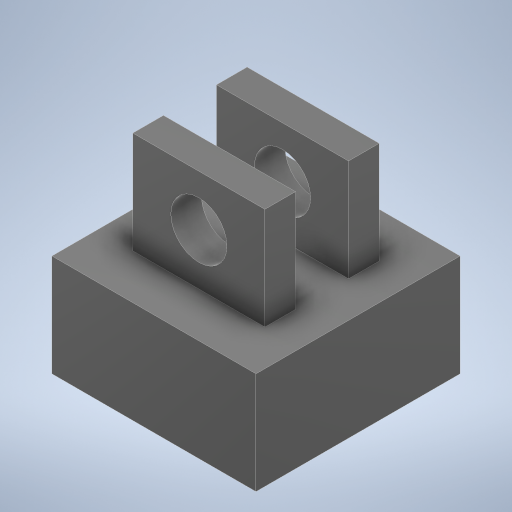
# Autodesk Inventor part: RollZ
Saved by Autodesk Inventor 2023 (Build 270158000, 158)
## iProperties
Created: 2023-10-26
Part Number: RollZ
Material: Thermoplastic Resin
Document SubType Name: Modeling
Designer: Mustapha
Density: 1.28 g/cm^3
Appearance: Smooth - Black
Mass: 5.5597 g
Surface Area: 24.3284 cm^2
Volume: 4.34352 cm^3
Author: Mustapha
Autodesk Inventor part; units mm, degrees
ref_plane "YZ Plane" through (0, 0, 0) normal (1, 0, 0) x (0, 1, 0)
ref_plane "XZ Plane" through (0, 0, 0) normal (0, 1, 0) x (-1, 0, 0)
ref_plane "XY Plane" through (0, 0, 0) normal (0, 0, 1) x (1, 0, 0)
sketch "Sketch1" plane through (0, 0, 0) normal (0, 1, 0) x (-1, 0, 0)
  line L0 (0, 0) -> (20, 0)
  line L1 (20, 0) -> (20, -20)
  line L2 (20, -20) -> (0, -20)
  line L3 (0, -20) -> (0, 0)
  point P0 (0, -10)
  point P1 (20, -10)
  dimension "d0" = 20
  dimension "d1" = 20
  constraints: 8 end point, 2 midpoint, 2 parallel, 1 horizontal, 1 perpendicular
  measures "d0" distance between parallel lines of L2 L0
  measures "d1" distance of point (0, -10) point (20, -10)
extrude "Extrusion1" add sketch "Sketch1" along normal blind 10
sketch "Sketch2" plane through (0, 0, 0) normal (0, -1, 0) x (1, 0, 0)
  circle A0 centre (-10, -10) radius 2.1511
  line L0 (-20, 0) -> (0, 0) projected
  line L1 (-13.8262, -12.1511) -> (-13.776, -7.7619)
  line L2 (-13.776, -7.7619) -> (-9.9498, -5.6108)
  line L3 (-9.9498, -5.6108) -> (-6.1738, -7.8489)
  line L4 (-6.1738, -7.8489) -> (-6.224, -12.2381)
  line L5 (-6.224, -12.2381) -> (-10.0502, -14.3892)
  line L6 (-10.0502, -14.3892) -> (-13.8262, -12.1511)
  dimension "d4" = 10
  constraints: 12 end point, 1 centre point, 1 coincident, 13 other
  measures "d4" distance from line of L0 A0.centre
extrude "Extrusion2" cut sketch "Sketch2" against normal blind 1 contours A0 | L1 L2 L3 L4 L5 L6
sketch "Sketch3" plane through (0, 1, 0) normal (0, -1, 0) x (1, 0, 0)
  circle A0 centre (-9.9498, -10) radius 3
  line L0 (-20, 0) -> (0, 0) projected
  point P0 (-10, 0)
  dimension "d7" = 6
  dimension "d8" = 10
  constraints: 1 centre point, 1 midpoint
  measures "d7" diameter of A0
  measures "d8" vertical distance of point (-10, 0) A0.centre
extrude "Extrusion3" cut sketch "Sketch3" against normal blind 8.5
sketch "Sketch4" plane through (0, 10, 0) normal (0, 1, 0) x (1, 0, 0)
  line L0 (0, 0) -> (0, 20) projected
  line L1 (-20, 20) -> (-20, 0) projected
  line L2 (0, 0) -> (-20, 20)
  line L3 (-20, 20) -> (-20, 0)
  line L4 (-20, 0) -> (0, 20)
  line L5 (0, 20) -> (0, 10)
  line L6 (0, 10) -> (-20, 10)
  line L7 (-20, 0) -> (0, 0) projected
  line L8 (-10, 0) -> (-10, 20)
  line L9 (-3.5295, 15.6) -> (-10, 15.6)
  line L10 (-10, 15.6) -> (-10, 12.6)
  line L11 (-10, 12.6) -> (-3.5295, 12.6)
  line L12 (-3.5295, 12.6) -> (-3.5295, 15.6)
  line L13 (-16.4705, 15.6) -> (-10, 15.6)
  line L14 (-10, 12.6) -> (-16.4705, 12.6)
  line L15 (-16.4705, 12.6) -> (-16.4705, 15.6)
  line L16 (-3.5295, 4.4) -> (-10, 4.4)
  line L17 (-10, 7.4) -> (-3.5295, 7.4)
  line L18 (-3.5295, 7.4) -> (-3.5295, 4.4)
  line L19 (-10, 7.4) -> (-16.4705, 7.4)
  line L20 (-16.4705, 7.4) -> (-16.4705, 4.4)
  line L21 (-16.4705, 4.4) -> (-10, 4.4)
  point P0 (-6.7648, 12.6)
  point P1 (-6.7648, 15.6)
  dimension "d11" = 3
  dimension "d18" = 5.2
  constraints: 38 end point, 8 symmetric about line, 4 midpoint, 3 parallel, 2 perpendicular, 1 collinear, 1 horizontal, 1 point on line, 1 vertical
  measures "d11" distance of point (-6.765, 12.6) point (-6.765, 15.6)
  measures "d18" diameter of L14 L6
extrude "Extrusion4" add sketch "Sketch4" along normal blind 10 contours L16 L8 L17 L2 | L2 L17 L18 L16 | L21 L4 L19 L8 | L9 L12 L11 L4 | L4 L11 L8 L9 | L14 L15 L13 L2 | L2 L13 L8 L14 | L4 L21 L20 L19
sketch "Sketch5" plane through (-3.5295, 10, -15.6) normal (0, 0, -1) x (-1, 0, 0)
  circle A0 centre (6.4705, 5) radius 2.75
  line L0 (0, 10) -> (12.941, 10) projected
  line L1 (16.4705, 0) -> (-3.5295, 0) projected
  line L2 (0, 0) -> (0, 10) projected
  line L3 (12.941, 0) -> (12.941, 10) projected
  point P0 (-3.5295, -10)
  dimension "d14" = 5.5
  dimension "d15" = 5
  dimension "d19" = 10
  dimension "d20" = 12.941
  constraints: 1 centre point
  measures "d14" diameter of A0
  measures "d15" distance from line of L0 A0.centre
  measures "d19" distance between parallel lines of L1 L0
  measures "d20" distance between parallel lines of L2 L3
extrude "Extrusion5" cut sketch "Sketch5" against normal blind 66.5 contours A0
body "Solid1"
